Autodesk Fusion 360 part; units mm, degrees
(part 2 of 5)
  spline S37 degree 5 poles (9.6613, 25.5009) (9.6619, 25.504) (9.6641, 25.5157) (9.6678, 25.5361) (9.673, 25.5652) (9.6795, 25.6029) (9.6866, 25.6464) (9.6934, 25.69) (9.6999, 25.7337) (9.7061, 25.7775) (9.7119, 25.8213) (9.7174, 25.8653) (9.7226, 25.9094) (9.7275, 25.9535) (9.7322, 25.9977) (9.7365, 26.042) (9.7407, 26.0863) (9.7445, 26.1308) (9.7481, 26.1753) (9.7514, 26.2199) (9.7545, 26.2645) (9.7573, 26.3092) (9.7599, 26.354) (9.7623, 26.3988) (9.7644, 26.4437) (9.7663, 26.4886) (9.7679, 26.5336) (9.7694, 26.5787) (9.7706, 26.6238) (9.7715, 26.669) (9.7723, 26.7142) (9.7728, 26.7595) (9.7732, 26.8048) (9.7733, 26.8502) (9.7732, 26.8956) (9.7729, 26.9411) (9.7724, 26.9866) (9.7716, 27.0321) (9.7707, 27.0777) (9.7696, 27.1234) (9.7683, 27.169) (9.7667, 27.2148) (9.765, 27.2605) (9.7631, 27.3063) (9.761, 27.3522) (9.7587, 27.3981) (9.7562, 27.444) (9.7535, 27.4899) (9.7506, 27.5359) (9.7476, 27.582) (9.7443, 27.628) (9.7409, 27.6741) (9.7373, 27.7202) (9.7335, 27.7664) (9.7295, 27.8126) (9.7254, 27.8588) (9.721, 27.9051) (9.7165, 27.9514) (9.7118, 27.9977) (9.7069, 28.044) (9.7019, 28.0904) (9.6967, 28.1368) (9.6923, 28.1739) (9.689, 28.2018) (9.6868, 28.2203) (9.6856, 28.2296) knots 0.13777296 0.13777296 0.13777296 0.13777296 0.13777296 0.13777296 0.14285714 0.15714286 0.17142857 0.18571429 0.2 0.21428571 0.22857143 0.24285714 0.25714286 0.27142857 0.28571429 0.3 0.31428571 0.32857143 0.34285714 0.35714286 0.37142857 0.38571429 0.4 0.41428571 0.42857143 0.44285714 0.45714286 0.47142857 0.48571429 0.5 0.51428571 0.52857143 0.54285714 0.55714286 0.57142857 0.58571429 0.6 0.61428571 0.62857143 0.64285714 0.65714286 0.67142857 0.68571429 0.7 0.71428571 0.72857143 0.74285714 0.75714286 0.77142857 0.78571429 0.8 0.81428571 0.82857143 0.84285714 0.85714286 0.87142857 0.88571429 0.9 0.91428571 0.92857143 0.94285714 0.95714286 0.97142857 0.98571429 1 1 1 1 1 1
  arc A19 (9.6856, 28.2296) -> (8.7571, 28.5313) centre (0, 0) ccw
  spline S38 degree 5 poles (8.7571, 28.5313) (8.7507, 28.5245) (8.738, 28.5108) (8.7189, 28.4902) (8.6936, 28.4627) (8.6621, 28.4282) (8.6308, 28.3937) (8.5996, 28.359) (8.5686, 28.3243) (8.5377, 28.2895) (8.507, 28.2547) (8.4765, 28.2197) (8.4461, 28.1847) (8.4159, 28.1496) (8.3859, 28.1144) (8.356, 28.0791) (8.3263, 28.0438) (8.2968, 28.0083) (8.2674, 27.9728) (8.2382, 27.9372) (8.2092, 27.9015) (8.1804, 27.8658) (8.1517, 27.8299) (8.1233, 27.794) (8.095, 27.758) (8.0669, 27.7219) (8.0389, 27.6857) (8.0112, 27.6494) (7.9837, 27.6131) (7.9563, 27.5766) (7.9291, 27.5401) (7.9022, 27.5035) (7.8754, 27.4668) (7.8488, 27.4301) (7.8224, 27.3932) (7.7963, 27.3563) (7.7703, 27.3192) (7.7445, 27.2821) (7.719, 27.2449) (7.6937, 27.2076) (7.6685, 27.1702) (7.6436, 27.1328) (7.619, 27.0952) (7.5945, 27.0576) (7.5703, 27.0198) (7.5463, 26.982) (7.5226, 26.9441) (7.4991, 26.906) (7.4758, 26.8679) (7.4528, 26.8297) (7.4301, 26.7914) (7.4076, 26.753) (7.3854, 26.7145) (7.3634, 26.6759) (7.3417, 26.6372) (7.3203, 26.5984) (7.2992, 26.5595) (7.2785, 26.5205) (7.258, 26.4813) (7.2379, 26.4421) (7.2181, 26.4027) (7.2012, 26.3683) (7.1883, 26.3418) (7.1794, 26.3231) (7.1742, 26.3123) (7.1729, 26.3095) knots -1 -1 -1 -1 -1 -1 -0.98571429 -0.97142857 -0.95714286 -0.94285714 -0.92857143 -0.91428571 -0.9 -0.88571429 -0.87142857 -0.85714286 -0.84285714 -0.82857143 -0.81428571 -0.8 -0.78571429 -0.77142857 -0.75714286 -0.74285714 -0.72857143 -0.71428571 -0.7 -0.68571429 -0.67142857 -0.65714286 -0.64285714 -0.62857143 -0.61428571 -0.6 -0.58571429 -0.57142857 -0.55714286 -0.54285714 -0.52857143 -0.51428571 -0.5 -0.48571429 -0.47142857 -0.45714286 -0.44285714 -0.42857143 -0.41428571 -0.4 -0.38571429 -0.37142857 -0.35714286 -0.34285714 -0.32857143 -0.31428571 -0.3 -0.28571429 -0.27142857 -0.25714286 -0.24285714 -0.22857143 -0.21428571 -0.2 -0.18571429 -0.17142857 -0.15714286 -0.14285714 -0.13777296 -0.13777296 -0.13777296 -0.13777296 -0.13777296 -0.13777296
  spline S39 degree 3 poles (6.941, 26.2019) (6.9661, 26.1952) (6.9924, 26.1935) (7.044, 26.2003) (7.0689, 26.2087) (7.1092, 26.2317) (7.1252, 26.2444) (7.1527, 26.2742) (7.1642, 26.2911) (7.1729, 26.3095) knots 0 0 0 0 0.007813 0.007813 0.015626 0.015626 0.021719 0.021719 0.027811 0.027811 0.027811 0.027811
  arc A20 (6.941, 26.2019) -> (6.1725, 26.3935) centre (0, 0) ccw
  spline S40 degree 3 poles (6.0183, 26.5974) (6.0171, 26.5714) (6.021, 26.5454) (6.0385, 26.4963) (6.052, 26.4737) (6.083, 26.4393) (6.0988, 26.4264) (6.1338, 26.4057) (6.1527, 26.3981) (6.1725, 26.3935) knots 0 0 0 0 0.007813 0.007813 0.015626 0.015626 0.021719 0.021719 0.027811 0.027811 0.027811 0.027811
  spline S41 degree 5 poles (6.0183, 26.5974) (6.0184, 26.6005) (6.0189, 26.6124) (6.0198, 26.6331) (6.0209, 26.6626) (6.0221, 26.7009) (6.0231, 26.745) (6.0238, 26.7891) (6.0241, 26.8332) (6.0241, 26.8774) (6.0237, 26.9217) (6.0231, 26.966) (6.0221, 27.0103) (6.0208, 27.0547) (6.0193, 27.0991) (6.0174, 27.1436) (6.0153, 27.1881) (6.013, 27.2326) (6.0103, 27.2772) (6.0074, 27.3218) (6.0043, 27.3665) (6.0009, 27.4111) (5.9972, 27.4558) (5.9933, 27.5005) (5.9891, 27.5453) (5.9847, 27.5901) (5.9801, 27.6348) (5.9752, 27.6797) (5.9702, 27.7245) (5.9648, 27.7694) (5.9593, 27.8143) (5.9535, 27.8592) (5.9475, 27.9041) (5.9413, 27.949) (5.9349, 27.994) (5.9283, 28.039) (5.9214, 28.084) (5.9144, 28.129) (5.9071, 28.174) (5.8997, 28.2191) (5.892, 28.2641) (5.8841, 28.3092) (5.8761, 28.3543) (5.8678, 28.3994) (5.8593, 28.4445) (5.8506, 28.4896) (5.8418, 28.5347) (5.8327, 28.5798) (5.8235, 28.625) (5.8141, 28.6701) (5.8044, 28.7153) (5.7946, 28.7605) (5.7846, 28.8056) (5.7744, 28.8508) (5.7641, 28.896) (5.7535, 28.9412) (5.7428, 28.9864) (5.7319, 29.0316) (5.7208, 29.0768) (5.7095, 29.122) (5.698, 29.1672) (5.6864, 29.2124) (5.677, 29.2486) (5.6698, 29.2758) (5.665, 29.2938) (5.6626, 29.3029) knots 0.13777296 0.13777296 0.13777296 0.13777296 0.13777296 0.13777296 0.14285714 0.15714286 0.17142857 0.18571429 0.2 0.21428571 0.22857143 0.24285714 0.25714286 0.27142857 0.28571429 0.3 0.31428571 0.32857143 0.34285714 0.35714286 0.37142857 0.38571429 0.4 0.41428571 0.42857143 0.44285714 0.45714286 0.47142857 0.48571429 0.5 0.51428571 0.52857143 0.54285714 0.55714286 0.57142857 0.58571429 0.6 0.61428571 0.62857143 0.64285714 0.65714286 0.67142857 0.68571429 0.7 0.71428571 0.72857143 0.74285714 0.75714286 0.77142857 0.78571429 0.8 0.81428571 0.82857143 0.84285714 0.85714286 0.87142857 0.88571429 0.9 0.91428571 0.92857143 0.94285714 0.95714286 0.97142857 0.98571429 1 1 1 1 1 1
  arc A21 (5.6626, 29.3029) -> (4.7011, 29.4724) centre (0, 0) ccw
  spline S42 degree 5 poles (4.7011, 29.4724) (4.6957, 29.4647) (4.685, 29.4494) (4.669, 29.4264) (4.6478, 29.3956) (4.6214, 29.3571) (4.5951, 29.3185) (4.5691, 29.2799) (4.5432, 29.2412) (4.5175, 29.2025) (4.4919, 29.1637) (4.4666, 29.1248) (4.4414, 29.0859) (4.4163, 29.0469) (4.3915, 29.0079) (4.3668, 28.9688) (4.3423, 28.9296) (4.318, 28.8904) (4.2939, 28.8512) (4.27, 28.8119) (4.2462, 28.7725) (4.2226, 28.7331) (4.1992, 28.6936) (4.176, 28.654) (4.153, 28.6144) (4.1302, 28.5748) (4.1076, 28.5351) (4.0852, 28.4953) (4.063, 28.4555) (4.0409, 28.4156) (4.0191, 28.3756) (3.9975, 28.3356) (3.9761, 28.2956) (3.9549, 28.2555) (3.9339, 28.2153) (3.9131, 28.1751) (3.8926, 28.1348) (3.8722, 28.0944) (3.8521, 28.054) (3.8322, 28.0136) (3.8125, 27.9731) (3.7931, 27.9325) (3.7739, 27.8919) (3.7549, 27.8512) (3.7362, 27.8104) (3.7177, 27.7696) (3.6995, 27.7288) (3.6815, 27.6879) (3.6638, 27.6469) (3.6463, 27.6058) (3.6291, 27.5647) (3.6122, 27.5236) (3.5955, 27.4824) (3.5792, 27.4411) (3.5631, 27.3997) (3.5473, 27.3583) (3.5318, 27.3169) (3.5167, 27.2753) (3.5019, 27.2337) (3.4875, 27.1921) (3.4733, 27.1503) (3.4613, 27.1139) (3.4523, 27.0858) (3.446, 27.0661) (3.4425, 27.0547) (3.4415, 27.0517) knots -1 -1 -1 -1 -1 -1 -0.98571429 -0.97142857 -0.95714286 -0.94285714 -0.92857143 -0.91428571 -0.9 -0.88571429 -0.87142857 -0.85714286 -0.84285714 -0.82857143 -0.81428571 -0.8 -0.78571429 -0.77142857 -0.75714286 -0.74285714 -0.72857143 -0.71428571 -0.7 -0.68571429 -0.67142857 -0.65714286 -0.64285714 -0.62857143 -0.61428571 -0.6 -0.58571429 -0.57142857 -0.55714286 -0.54285714 -0.52857143 -0.51428571 -0.5 -0.48571429 -0.47142857 -0.45714286 -0.44285714 -0.42857143 -0.41428571 -0.4 -0.38571429 -0.37142857 -0.35714286 -0.34285714 -0.32857143 -0.31428571 -0.3 -0.28571429 -0.27142857 -0.25714286 -0.24285714 -0.22857143 -0.21428571 -0.2 -0.18571429 -0.17142857 -0.15714286 -0.14285714 -0.13777296 -0.13777296 -0.13777296 -0.13777296 -0.13777296 -0.13777296
  spline S43 degree 3 poles (3.2268, 26.9129) (3.2527, 26.9098) (3.2789, 26.9117) (3.3291, 26.9256) (3.3526, 26.9374) (3.3892, 26.9658) (3.4033, 26.9806) (3.4265, 27.014) (3.4355, 27.0323) (3.4415, 27.0517) knots 0 0 0 0 0.007813 0.007813 0.015626 0.015626 0.021719 0.021719 0.027811 0.027811 0.027811 0.027811
  arc A22 (3.2268, 26.9129) -> (2.4392, 26.9956) centre (0, 0) ccw
  spline S44 degree 3 poles (2.2581, 27.1761) (2.2605, 27.1502) (2.268, 27.125) (2.2922, 27.0788) (2.3087, 27.0584) (2.3442, 27.0286) (2.3616, 27.018) (2.3991, 27.0024) (2.419, 26.9975) (2.4392, 26.9956) knots 0 0 0 0 0.007813 0.007813 0.015626 0.015626 0.021719 0.021719 0.027811 0.027811 0.027811 0.027811
  spline S45 degree 5 poles (2.2581, 27.1761) (2.2578, 27.1792) (2.2566, 27.1911) (2.2546, 27.2117) (2.2516, 27.2411) (2.2474, 27.2792) (2.2423, 27.3229) (2.2368, 27.3667) (2.231, 27.4105) (2.2248, 27.4542) (2.2183, 27.498) (2.2115, 27.5418) (2.2044, 27.5856) (2.1969, 27.6294) (2.1892, 27.6731) (2.1812, 27.7169) (2.1729, 27.7607) (2.1644, 27.8045) (2.1556, 27.8482) (2.1465, 27.892) (2.1372, 27.9358) (2.1276, 27.9795) (2.1177, 28.0233) (2.1076, 28.067) (2.0973, 28.1107) (2.0867, 28.1545) (2.0759, 28.1982) (2.0648, 28.2419) (2.0536, 28.2856) (2.042, 28.3293) (2.0303, 28.373) (2.0183, 28.4166) (2.0062, 28.4603) (1.9938, 28.5039) (1.9812, 28.5476) (1.9683, 28.5912) (1.9553, 28.6348) (1.942, 28.6784) (1.9286, 28.7219) (1.9149, 28.7655) (1.9011, 28.8091) (1.887, 28.8526) (1.8727, 28.8961) (1.8583, 28.9396) (1.8436, 28.9831) (1.8287, 29.0266) (1.8137, 29.07) (1.7984, 29.1135) (1.783, 29.1569) (1.7674, 29.2003) (1.7515, 29.2437) (1.7355, 29.287) (1.7194, 29.3304) (1.703, 29.3737) (1.6864, 29.417) (1.6697, 29.4603) (1.6528, 29.5036) (1.6357, 29.5468) (1.6184, 29.59) (1.6009, 29.6332) (1.5833, 29.6764) (1.5655, 29.7196) (1.5511, 29.7541) (1.5402, 29.7799) (1.5329, 29.7972) (1.5293, 29.8058) knots 0.13777296 0.13777296 0.13777296 0.13777296 0.13777296 0.13777296 0.14285714 0.15714286 0.17142857 0.18571429 0.2 0.21428571 0.22857143 0.24285714 0.25714286 0.27142857 0.28571429 0.3 0.31428571 0.32857143 0.34285714 0.35714286 0.37142857 0.38571429 0.4 0.41428571 0.42857143 0.44285714 0.45714286 0.47142857 0.48571429 0.5 0.51428571 0.52857143 0.54285714 0.55714286 0.57142857 0.58571429 0.6 0.61428571 0.62857143 0.64285714 0.65714286 0.67142857 0.68571429 0.7 0.71428571 0.72857143 0.74285714 0.75714286 0.77142857 0.78571429 0.8 0.81428571 0.82857143 0.84285714 0.85714286 0.87142857 0.88571429 0.9 0.91428571 0.92857143 0.94285714 0.95714286 0.97142857 0.98571429 1 1 1 1 1 1
  arc A23 (1.5293, 29.8058) -> (0.5536, 29.8399) centre (0, 0) ccw
  spline S46 degree 5 poles (0.5536, 29.8399) (0.5493, 29.8315) (0.5409, 29.8148) (0.5282, 29.7898) (0.5115, 29.7564) (0.4907, 29.7145) (0.4701, 29.6727) (0.4497, 29.6308) (0.4294, 29.5889) (0.4093, 29.547) (0.3894, 29.505) (0.3697, 29.463) (0.3502, 29.4209) (0.3308, 29.3789) (0.3116, 29.3368) (0.2927, 29.2946) (0.2739, 29.2524) (0.2552, 29.2102) (0.2368, 29.168) (0.2186, 29.1257) (0.2005, 29.0834) (0.1827, 29.0411) (0.165, 28.9987) (0.1475, 28.9564) (0.1303, 28.9139) (0.1132, 28.8715) (0.0963, 28.829) (0.0797, 28.7865) (0.0632, 28.744) (0.0469, 28.7014) (0.0309, 28.6588) (0.015, 28.6162) (-0.0006, 28.5736) (-0.016, 28.5309) (-0.0312, 28.4882) (-0.0462, 28.4455) (-0.0609, 28.4027) (-0.0754, 28.3599) (-0.0897, 28.3171) (-0.1038, 28.2743) (-0.1177, 28.2314) (-0.1313, 28.1886) (-0.1446, 28.1457) (-0.1578, 28.1027) (-0.1706, 28.0598) (-0.1833, 28.0168) (-0.1956, 27.9738) (-0.2077, 27.9308) (-0.2196, 27.8877) (-0.2312, 27.8446) (-0.2425, 27.8016) (-0.2535, 27.7584) (-0.2643, 27.7153) (-0.2747, 27.6721) (-0.2849, 27.629) (-0.2948, 27.5858) (-0.3043, 27.5426) (-0.3135, 27.4993) (-0.3224, 27.4561) (-0.3309, 27.4128) (-0.3391, 27.3695) (-0.3459, 27.3318) (-0.3509, 27.3027) (-0.3544, 27.2823) (-0.3563, 27.2705) (-0.3568, 27.2674) knots -1 -1 -1 -1 -1 -1 -0.98571429 -0.97142857 -0.95714286 -0.94285714 -0.92857143 -0.91428571 -0.9 -0.88571429 -0.87142857 -0.85714286 -0.84285714 -0.82857143 -0.81428571 -0.8 -0.78571429 -0.77142857 -0.75714286 -0.74285714 -0.72857143 -0.71428571 -0.7 -0.68571429 -0.67142857 -0.65714286 -0.64285714 -0.62857143 -0.61428571 -0.6 -0.58571429 -0.57142857 -0.55714286 -0.54285714 -0.52857143 -0.51428571 -0.5 -0.48571429 -0.47142857 -0.45714286 -0.44285714 -0.42857143 -0.41428571 -0.4 -0.38571429 -0.37142857 -0.35714286 -0.34285714 -0.32857143 -0.31428571 -0.3 -0.28571429 -0.27142857 -0.25714286 -0.24285714 -0.22857143 -0.21428571 -0.2 -0.18571429 -0.17142857 -0.15714286 -0.14285714 -0.13777296 -0.13777296 -0.13777296 -0.13777296 -0.13777296 -0.13777296
  spline S47 degree 3 poles (-0.5501, 27.1) (-0.5241, 27.1006) (-0.4984, 27.1062) (-0.4506, 27.1269) (-0.429, 27.1419) (-0.3967, 27.1751) (-0.3848, 27.1917) (-0.3665, 27.228) (-0.3602, 27.2474) (-0.3568, 27.2674) knots 0 0 0 0 0.007813 0.007813 0.015626 0.015626 0.021719 0.021719 0.027811 0.027811 0.027811 0.027811
  arc A24 (-0.5501, 27.1) -> (-1.3416, 27.0724) centre (0, 0) ccw
  spline S48 degree 3 poles (-1.5461, 27.2259) (-1.5401, 27.2006) (-1.5292, 27.1766) (-1.4988, 27.1343) (-1.4796, 27.1163) (-1.4403, 27.0918) (-1.4215, 27.0837) (-1.3822, 27.0735) (-1.3619, 27.0714) (-1.3416, 27.0724) knots 0 0 0 0 0.007813 0.007813 0.015626 0.015626 0.021719 0.021719 0.027811 0.027811 0.027811 0.027811
  spline S49 degree 5 poles (-1.5461, 27.2259) (-1.5468, 27.2289) (-1.5496, 27.2405) (-1.5545, 27.2607) (-1.5615, 27.2893) (-1.571, 27.3265) (-1.5821, 27.3691) (-1.5937, 27.4117) (-1.6055, 27.4542) (-1.6177, 27.4967) (-1.6302, 27.5391) (-1.6431, 27.5815) (-1.6563, 27.6239) (-1.6697, 27.6662) (-1.6834, 27.7085) (-1.6975, 27.7507) (-1.7117, 27.7929) (-1.7263, 27.8351) (-1.7411, 27.8772) (-1.7562, 27.9193) (-1.7715, 27.9613) (-1.7871, 28.0033) (-1.803, 28.0453) (-1.8191, 28.0872) (-1.8354, 28.129) (-1.852, 28.1709) (-1.8687, 28.2127) (-1.8858, 28.2544) (-1.903, 28.2961) (-1.9205, 28.3378) (-1.9382, 28.3794) (-1.9561, 28.421) (-1.9743, 28.4625) (-1.9926, 28.504) (-2.0112, 28.5455) (-2.03, 28.5869) (-2.0489, 28.6282) (-2.0681, 28.6696) (-2.0875, 28.7108) (-2.1071, 28.7521) (-2.1269, 28.7933) (-2.1469, 28.8344) (-2.1671, 28.8755) (-2.1874, 28.9166) (-2.208, 28.9576) (-2.2288, 28.9986) (-2.2497, 29.0395) (-2.2709, 29.0804) (-2.2922, 29.1213) (-2.3137, 29.1621) (-2.3354, 29.2028) (-2.3573, 29.2436) (-2.3794, 29.2842) (-2.4016, 29.3248) (-2.424, 29.3654) (-2.4466, 29.406) (-2.4694, 29.4464) (-2.4924, 29.4869) (-2.5155, 29.5273) (-2.5388, 29.5676) (-2.5623, 29.6079) (-2.5859, 29.6482) (-2.605, 29.6804) (-2.6193, 29.7045) (-2.6289, 29.7205) (-2.6338, 29.7286) knots 0.13777296 0.13777296 0.13777296 0.13777296 0.13777296 0.13777296 0.14285714 0.15714286 0.17142857 0.18571429 0.2 0.21428571 0.22857143 0.24285714 0.25714286 0.27142857 0.28571429 0.3 0.31428571 0.32857143 0.34285714 0.35714286 0.37142857 0.38571429 0.4 0.41428571 0.42857143 0.44285714 0.45714286 0.47142857 0.48571429 0.5 0.51428571 0.52857143 0.54285714 0.55714286 0.57142857 0.58571429 0.6 0.61428571 0.62857143 0.64285714 0.65714286 0.67142857 0.68571429 0.7 0.71428571 0.72857143 0.74285714 0.75714286 0.77142857 0.78571429 0.8 0.81428571 0.82857143 0.84285714 0.85714286 0.87142857 0.88571429 0.9 0.91428571 0.92857143 0.94285714 0.95714286 0.97142857 0.98571429 1 1 1 1 1 1
  arc A25 (-2.6338, 29.7286) -> (-3.6047, 29.6265) centre (0, 0) ccw
  spline S50 degree 5 poles (-3.6047, 29.6265) (-3.6078, 29.6177) (-3.6138, 29.5999) (-3.6229, 29.5734) (-3.6348, 29.538) (-3.6496, 29.4937) (-3.6641, 29.4494) (-3.6785, 29.405) (-3.6928, 29.3607) (-3.7068, 29.3164) (-3.7207, 29.2721) (-3.7343, 29.2277) (-3.7478, 29.1834) (-3.7611, 29.139) (-3.7743, 29.0946) (-3.7872, 29.0502) (-3.8, 29.0059) (-3.8125, 28.9615) (-3.8249, 28.9171) (-3.8371, 28.8727) (-3.8491, 28.8283) (-3.8609, 28.7839) (-3.8725, 28.7395) (-3.8838, 28.6951) (-3.895, 28.6507) (-3.906, 28.6063) (-3.9168, 28.5619) (-3.9274, 28.5175) (-3.9378, 28.473) (-3.948, 28.4286) (-3.958, 28.3842) (-3.9677, 28.3398) (-3.9772, 28.2954) (-3.9866, 28.251) (-3.9957, 28.2066) (-4.0046, 28.1622) (-4.0132, 28.1178) (-4.0217, 28.0734) (-4.0299, 28.0291) (-4.0378, 27.9847) (-4.0456, 27.9403) (-4.0531, 27.896) (-4.0603, 27.8516) (-4.0674, 27.8073) (-4.0741, 27.7629) (-4.0807, 27.7186) (-4.0869, 27.6743) (-4.0929, 27.63) (-4.0987, 27.5858) (-4.1041, 27.5415) (-4.1093, 27.4972) (-4.1143, 27.453) (-4.1189, 27.4088) (-4.1233, 27.3646) (-4.1273, 27.3204) (-4.1311, 27.2763) (-4.1345, 27.2322) (-4.1376, 27.1881) (-4.1404, 27.144) (-4.1428, 27.1) (-4.1449, 27.0559) (-4.1464, 27.0176) (-4.1473, 26.9881) (-4.1479, 26.9674) (-4.1482, 26.9555) (-4.1483, 26.9524) knots -1 -1 -1 -1 -1 -1 -0.98571429 -0.97142857 -0.95714286 -0.94285714 -0.92857143 -0.91428571 -0.9 -0.88571429 -0.87142857 -0.85714286 -0.84285714 -0.82857143 -0.81428571 -0.8 -0.78571429 -0.77142857 -0.75714286 -0.74285714 -0.72857143 -0.71428571 -0.7 -0.68571429 -0.67142857 -0.65714286 -0.64285714 -0.62857143 -0.61428571 -0.6 -0.58571429 -0.57142857 -0.55714286 -0.54285714 -0.52857143 -0.51428571 -0.5 -0.48571429 -0.47142857 -0.45714286 -0.44285714 -0.42857143 -0.41428571 -0.4 -0.38571429 -0.37142857 -0.35714286 -0.34285714 -0.32857143 -0.31428571 -0.3 -0.28571429 -0.27142857 -0.25714286 -0.24285714 -0.22857143 -0.21428571 -0.2 -0.18571429 -0.17142857 -0.15714286 -0.14285714 -0.13777296 -0.13777296 -0.13777296 -0.13777296 -0.13777296 -0.13777296
  spline S51 degree 3 poles (-4.3164, 26.7597) (-4.2906, 26.7639) (-4.266, 26.773) (-4.2216, 26.8002) (-4.2022, 26.818) (-4.1748, 26.8554) (-4.1654, 26.8735) (-4.1523, 26.912) (-4.1487, 26.9321) (-4.1483, 26.9524) knots 0 0 0 0 0.007813 0.007813 0.015626 0.015626 0.021719 0.021719 0.027811 0.027811 0.027811 0.027811
  arc A26 (-4.3164, 26.7597) -> (-5.0963, 26.6222) centre (0, 0) ccw
  spline S52 degree 3 poles (-5.3202, 26.7458) (-5.3107, 26.7215) (-5.2965, 26.6993) (-5.2606, 26.6617) (-5.2391, 26.6465) (-5.1967, 26.6277) (-5.177, 26.6223) (-5.1367, 26.6176) (-5.1163, 26.6184) (-5.0963, 26.6222) knots 0 0 0 0 0.007813 0.007813 0.015626 0.015626 0.021719 0.021719 0.027811 0.027811 0.027811 0.027811
  spline S53 degree 5 poles (-5.3202, 26.7458) (-5.3213, 26.7487) (-5.3257, 26.7598) (-5.3333, 26.779) (-5.3443, 26.8064) (-5.3588, 26.8419) (-5.3758, 26.8825) (-5.3931, 26.9231) (-5.4108, 26.9636) (-5.4288, 27.004) (-5.4471, 27.0442) (-5.4657, 27.0844) (-5.4846, 27.1246) (-5.5039, 27.1646) (-5.5233, 27.2046) (-5.5431, 27.2444) (-5.5631, 27.2842) (-5.5834, 27.324) (-5.6039, 27.3636) (-5.6247, 27.4032) (-5.6458, 27.4427) (-5.667, 27.4821) (-5.6886, 27.5214) (-5.7103, 27.5607) (-5.7323, 27.5999) (-5.7546, 27.639) (-5.777, 27.678) (-5.7997, 27.717) (-5.8226, 27.7559) (-5.8457, 27.7947) (-5.869, 27.8335) (-5.8925, 27.8721) (-5.9163, 27.9107) (-5.9402, 27.9493) (-5.9644, 27.9877) (-5.9887, 28.0261) (-6.0133, 28.0645) (-6.038, 28.1027) (-6.063, 28.1409) (-6.0881, 28.179) (-6.1134, 28.2171) (-6.139, 28.255) (-6.1647, 28.2929) (-6.1906, 28.3308) (-6.2167, 28.3685) (-6.2429, 28.4062) (-6.2694, 28.4438) (-6.296, 28.4814) (-6.3228, 28.5189) (-6.3498, 28.5563) (-6.377, 28.5936) (-6.4043, 28.6309) (-6.4318, 28.6681) (-6.4595, 28.7052) (-6.4873, 28.7423) (-6.5154, 28.7793) (-6.5435, 28.8162) (-6.5719, 28.8531) (-6.6004, 28.8898) (-6.6291, 28.9266) (-6.658, 28.9632) (-6.687, 28.9998) (-6.7103, 29.029) (-6.7279, 29.0508) (-6.7397, 29.0654) (-6.7455, 29.0727) knots 0.13777296 0.13777296 0.13777296 0.13777296 0.13777296 0.13777296 0.14285714 0.15714286 0.17142857 0.18571429 0.2 0.21428571 0.22857143 0.24285714 0.25714286 0.27142857 0.28571429 0.3 0.31428571 0.32857143 0.34285714 0.35714286 0.37142857 0.38571429 0.4 0.41428571 0.42857143 0.44285714 0.45714286 0.47142857 0.48571429 0.5 0.51428571 0.52857143 0.54285714 0.55714286 0.57142857 0.58571429 0.6 0.61428571 0.62857143 0.64285714 0.65714286 0.67142857 0.68571429 0.7 0.71428571 0.72857143 0.74285714 0.75714286 0.77142857 0.78571429 0.8 0.81428571 0.82857143 0.84285714 0.85714286 0.87142857 0.88571429 0.9 0.91428571 0.92857143 0.94285714 0.95714286 0.97142857 0.98571429 1 1 1 1 1 1
  arc A27 (-6.7455, 29.0727) -> (-7.6928, 28.8365) centre (0, 0) ccw
  spline S54 degree 5 poles (-7.6928, 28.8365) (-7.6946, 28.8273) (-7.6982, 28.8089) (-7.7034, 28.7814) (-7.7103, 28.7446) (-7.7188, 28.6987) (-7.727, 28.6528) (-7.7351, 28.6069) (-7.743, 28.5611) (-7.7508, 28.5152) (-7.7583, 28.4694) (-7.7657, 28.4235) (-7.7729, 28.3777) (-7.7799, 28.332) (-7.7867, 28.2862) (-7.7934, 28.2405) (-7.7998, 28.1947) (-7.8061, 28.149) (-7.8122, 28.1034) (-7.818, 28.0577) (-7.8237, 28.0121) (-7.8292, 27.9665) (-7.8345, 27.9209) (-7.8396, 27.8753) (-7.8445, 27.8298) (-7.8493, 27.7843) (-7.8538, 27.7388) (-7.8581, 27.6933) (-7.8622, 27.6479) (-7.8661, 27.6025) (-7.8698, 27.5571) (-7.8732, 27.5118) (-7.8765, 27.4665) (-7.8796, 27.4212) (-7.8824, 27.376) (-7.885, 27.3308) (-7.8874, 27.2856) (-7.8896, 27.2405) (-7.8915, 27.1954) (-7.8933, 27.1504) (-7.8947, 27.1054) (-7.896, 27.0604) (-7.897, 27.0155) (-7.8978, 26.9706) (-7.8983, 26.9257) (-7.8986, 26.881) (-7.8987, 26.8362) (-7.8985, 26.7915) (-7.898, 26.7469) (-7.8972, 26.7023) (-7.8962, 26.6577) (-7.8949, 26.6132) (-7.8934, 26.5688) (-7.8916, 26.5245) (-7.8894, 26.4801) (-7.887, 26.4359) (-7.8843, 26.3917) (-7.8812, 26.3476) (-7.8778, 26.3036) (-7.874, 26.2597) (-7.87, 26.2158) (-7.8661, 26.1776) (-7.863, 26.1483) (-7.8607, 26.1277) (-7.8593, 26.1159) (-7.8589, 26.1128) knots -1 -1 -1 -1 -1 -1 -0.98571429 -0.97142857 -0.95714286 -0.94285714 -0.92857143 -0.91428571 -0.9 -0.88571429 -0.87142857 -0.85714286 -0.84285714 -0.82857143 -0.81428571 -0.8 -0.78571429 -0.77142857 -0.75714286 -0.74285714 -0.72857143 -0.71428571 -0.7 -0.68571429 -0.67142857 -0.65714286 -0.64285714 -0.62857143 -0.61428571 -0.6 -0.58571429 -0.57142857 -0.55714286 -0.54285714 -0.52857143 -0.51428571 -0.5 -0.48571429 -0.47142857 -0.45714286 -0.44285714 -0.42857143 -0.41428571 -0.4 -0.38571429 -0.37142857 -0.35714286 -0.34285714 -0.32857143 -0.31428571 -0.3 -0.28571429 -0.27142857 -0.25714286 -0.24285714 -0.22857143 -0.21428571 -0.2 -0.18571429 -0.17142857 -0.15714286 -0.14285714 -0.13777296 -0.13777296 -0.13777296 -0.13777296 -0.13777296 -0.13777296
  spline S55 degree 3 poles (-7.9986, 25.8986) (-7.9737, 25.9063) (-7.9506, 25.9187) (-7.9104, 25.9519) (-7.8937, 25.9722) (-7.8718, 26.013) (-7.8649, 26.0323) (-7.8573, 26.0722) (-7.8566, 26.0926) (-7.8589, 26.1128) knots 0 0 0 0 0.007813 0.007813 0.015626 0.015626 0.021719 0.021719 0.027811 0.027811 0.027811 0.027811
  arc A28 (-7.9986, 25.8986) -> (-8.7518, 25.6538) centre (0, 0) ccw
  spline S56 degree 3 poles (-8.9907, 25.745) (-8.9779, 25.7223) (-8.9608, 25.7024) (-8.92, 25.6701) (-8.8966, 25.6581) (-8.852, 25.6453) (-8.8318, 25.6427) (-8.7911, 25.6437) (-8.771, 25.6473) (-8.7518, 25.6538) knots 0 0 0 0 0.007813 0.007813 0.015626 0.015626 0.021719 0.021719 0.027811 0.027811 0.027811 0.027811
  spline S57 degree 5 poles (-8.9907, 25.745) (-8.9922, 25.7478) (-8.9981, 25.7581) (-9.0083, 25.7762) (-9.023, 25.8017) (-9.0423, 25.8349) (-9.0648, 25.8728) (-9.0876, 25.9105) (-9.1107, 25.9481) (-9.1342, 25.9856) (-9.1579, 26.023) (-9.1819, 26.0602) (-9.2063, 26.0973) (-9.2309, 26.1342) (-9.2557, 26.1711) (-9.2808, 26.2078) (-9.3062, 26.2445) (-9.3318, 26.281) (-9.3577, 26.3174) (-9.3838, 26.3537) (-9.4101, 26.3898) (-9.4367, 26.4259) (-9.4635, 26.4619) (-9.4905, 26.4977) (-9.5177, 26.5335) (-9.5452, 26.5691) (-9.5728, 26.6047) (-9.6007, 26.6401) (-9.6288, 26.6754) (-9.6571, 26.7107) (-9.6855, 26.7458) (-9.7142, 26.7808) (-9.7431, 26.8157) (-9.7722, 26.8506) (-9.8015, 26.8853) (-9.8309, 26.9199) (-9.8606, 26.9545) (-9.8904, 26.9889) (-9.9204, 27.0232) (-9.9506, 27.0575) (-9.981, 27.0916) (-10.0116, 27.1257) (-10.0423, 27.1596) (-10.0732, 27.1935) (-10.1043, 27.2272) (-10.1355, 27.2609) (-10.167, 27.2945) (-10.1986, 27.328) (-10.2303, 27.3613) (-10.2623, 27.3946) (-10.2944, 27.4278) (-10.3266, 27.4609) (-10.359, 27.494) (-10.3916, 27.5269) (-10.4243, 27.5597) (-10.4572, 27.5924) (-10.4903, 27.6251) (-10.5235, 27.6576) (-10.5569, 27.6901) (-10.5904, 27.7224) (-10.6241, 27.7547) (-10.6579, 27.7869) (-10.6851, 27.8126) (-10.7055, 27.8318) (-10.7192, 27.8446) (-10.726, 27.851) knots 0.13777296 0.13777296 0.13777296 0.13777296 0.13777296 0.13777296 0.14285714 0.15714286 0.17142857 0.18571429 0.2 0.21428571 0.22857143 0.24285714 0.25714286 0.27142857 0.28571429 0.3 0.31428571 0.32857143 0.34285714 0.35714286 0.37142857 0.38571429 0.4 0.41428571 0.42857143 0.44285714 0.45714286 0.47142857 0.48571429 0.5 0.51428571 0.52857143 0.54285714 0.55714286 0.57142857 0.58571429 0.6 0.61428571 0.62857143 0.64285714 0.65714286 0.67142857 0.68571429 0.7 0.71428571 0.72857143 0.74285714 0.75714286 0.77142857 0.78571429 0.8 0.81428571 0.82857143 0.84285714 0.85714286 0.87142857 0.88571429 0.9 0.91428571 0.92857143 0.94285714 0.95714286 0.97142857 0.98571429 1 1 1 1 1 1
  arc A29 (-10.726, 27.851) -> (-11.6312, 27.4852) centre (0, 0) ccw
  spline S58 degree 5 poles (-11.6312, 27.4852) (-11.6317, 27.4759) (-11.6327, 27.4572) (-11.634, 27.4292) (-11.6358, 27.3918) (-11.6377, 27.3452) (-11.6395, 27.2986) (-11.6412, 27.252) (-11.6426, 27.2055) (-11.6439, 27.159) (-11.645, 27.1125) (-11.6459, 27.0662) (-11.6467, 27.0198) (-11.6472, 26.9735) (-11.6476, 26.9272) (-11.6478, 26.881) (-11.6479, 26.8348) (-11.6477, 26.7887) (-11.6474, 26.7426) (-11.6468, 26.6966) (-11.6461, 26.6506) (-11.6452, 26.6047) (-11.6441, 26.5588) (-11.6428, 26.513) (-11.6414, 26.4672) (-11.6397, 26.4215) (-11.6378, 26.3758) (-11.6358, 26.3302) (-11.6335, 26.2846) (-11.631, 26.2391) (-11.6284, 26.1937) (-11.6255, 26.1483) (-11.6224, 26.103) (-11.6192, 26.0578) (-11.6157, 26.0126) (-11.612, 25.9674) (-11.6081, 25.9224) (-11.6039, 25.8774) (-11.5996, 25.8325) (-11.595, 25.7876) (-11.5902, 25.7428) (-11.5852, 25.6981) (-11.58, 25.6535) (-11.5745, 25.6089) (-11.5688, 25.5645) (-11.5629, 25.5201) (-11.5567, 25.4758) (-11.5502, 25.4315) (-11.5436, 25.3874) (-11.5366, 25.3433) (-11.5294, 25.2994) (-11.522, 25.2555) (-11.5142, 25.2117) (-11.5063, 25.168) (-11.498, 25.1244) (-11.4894, 25.081) (-11.4806, 25.0376) (-11.4714, 24.9944) (-11.4619, 24.9512) (-11.4521, 24.9082) (-11.4419, 24.8654) (-11.4328, 24.8281) (-11.4256, 24.7995) (-11.4204, 24.7794) (-11.4174, 24.7679) (-11.4167, 24.7649) knots -1 -1 -1 -1 -1 -1 -0.98571429 -0.97142857 -0.95714286 -0.94285714 -0.92857143 -0.91428571 -0.9 -0.88571429 -0.87142857 -0.85714286 -0.84285714 -0.82857143 -0.81428571 -0.8 -0.78571429 -0.77142857 -0.75714286 -0.74285714 -0.72857143 -0.71428571 -0.7 -0.68571429 -0.67142857 -0.65714286 -0.64285714 -0.62857143 -0.61428571 -0.6 -0.58571429 -0.57142857 -0.55714286 -0.54285714 -0.52857143 -0.51428571 -0.5 -0.48571429 -0.47142857 -0.45714286 -0.44285714 -0.42857143 -0.41428571 -0.4 -0.38571429 -0.37142857 -0.35714286 -0.34285714 -0.32857143 -0.31428571 -0.3 -0.28571429 -0.27142857 -0.25714286 -0.24285714 -0.22857143 -0.21428571 -0.2 -0.18571429 -0.17142857 -0.15714286 -0.14285714 -0.13777296 -0.13777296 -0.13777296 -0.13777296 -0.13777296 -0.13777296
  spline S59 degree 3 poles (-11.5251, 24.5334) (-11.5016, 24.5444) (-11.4804, 24.56) (-11.4452, 24.5984) (-11.4315, 24.6208) (-11.4155, 24.6643) (-11.4114, 24.6843) (-11.4094, 24.7249) (-11.4115, 24.7452) (-11.4167, 24.7649) knots 0 0 0 0 0.007813 0.007813 0.015626 0.015626 0.021719 0.021719 0.027811 0.027811 0.027811 0.027811
  arc A30 (-11.5251, 24.5334) -> (-12.237, 24.1862) centre (0, 0) ccw
  spline S60 degree 3 poles (-12.4862, 24.2432) (-12.4704, 24.2225) (-12.4507, 24.2051) (-12.4057, 24.1788) (-12.3809, 24.1702) (-12.335, 24.1637) (-12.3146, 24.164) (-12.2745, 24.1706) (-12.2551, 24.177) (-12.237, 24.1862) knots 0 0 0 0 0.007813 0.007813 0.015626 0.015626 0.021719 0.021719 0.027811 0.027811 0.027811 0.027811
  spline S61 degree 5 poles (-12.4862, 24.2432) (-12.4881, 24.2457) (-12.4953, 24.2552) (-12.508, 24.2716) (-12.5261, 24.2949) (-12.5498, 24.325) (-12.5774, 24.3594) (-12.6052, 24.3936) (-12.6333, 24.4276) (-12.6618, 24.4615) (-12.6905, 24.4952) (-12.7195, 24.5287) (-12.7487, 24.562) (-12.7782, 24.5952) (-12.808, 24.6283) (-12.8379, 24.6611) (-12.8682, 24.6939) (-12.8986, 24.7265) (-12.9293, 24.7589) (-12.9602, 24.7912) (-12.9913, 24.8234) (-13.0226, 24.8554) (-13.0541, 24.8873) (-13.0859, 24.919) (-13.1178, 24.9506) (-13.15, 24.9821) (-13.1823, 25.0135) (-13.2148, 25.0447) (-13.2476, 25.0758) (-13.2805, 25.1067) (-13.3136, 25.1375) (-13.3469, 25.1682) (-13.3803, 25.1988) (-13.414, 25.2292) (-13.4478, 25.2595) (-13.4818, 25.2897) (-13.5159, 25.3198) (-13.5503, 25.3498) (-13.5848, 25.3796) (-13.6195, 25.4093) (-13.6543, 25.4389) (-13.6893, 25.4683) (-13.7245, 25.4977) (-13.7598, 25.5269) (-13.7953, 25.556) (-13.8309, 25.585) (-13.8667, 25.6139) (-13.9026, 25.6426) (-13.9387, 25.6713) (-13.975, 25.6998) (-14.0114, 25.7282) (-14.0479, 25.7565) (-14.0846, 25.7847) (-14.1215, 25.8128) (-14.1585, 25.8407) (-14.1956, 25.8685) (-14.2329, 25.8963) (-14.2703, 25.9239) (-14.3079, 25.9514) (-14.3455, 25.9788) (-14.3834, 26.006) (-14.4214, 26.0332) (-14.4518, 26.0548) (-14.4748, 26.071) (-14.4901, 26.0818) (-14.4977, 26.0871) knots 0.13777296 0.13777296 0.13777296 0.13777296 0.13777296 0.13777296 0.14285714 0.15714286 0.17142857 0.18571429 0.2 0.21428571 0.22857143 0.24285714 0.25714286 0.27142857 0.28571429 0.3 0.31428571 0.32857143 0.34285714 0.35714286 0.37142857 0.38571429 0.4 0.41428571 0.42857143 0.44285714 0.45714286 0.47142857 0.48571429 0.5 0.51428571 0.52857143 0.54285714 0.55714286 0.57142857 0.58571429 0.6 0.61428571 0.62857143 0.64285714 0.65714286 0.67142857 0.68571429 0.7 0.71428571 0.72857143 0.74285714 0.75714286 0.77142857 0.78571429 0.8 0.81428571 0.82857143 0.84285714 0.85714286 0.87142857 0.88571429 0.9 0.91428571 0.92857143 0.94285714 0.95714286 0.97142857 0.98571429 1 1 1 1 1 1
  arc A31 (-14.4977, 26.0871) -> (-15.3433, 25.599) centre (0, 0) ccw
  spline S62 degree 5 poles (-15.3433, 25.599) (-15.3424, 25.5897) (-15.3408, 25.571) (-15.3382, 25.5431) (-15.3347, 25.5059) (-15.3302, 25.4594) (-15.3255, 25.413) (-15.3206, 25.3666) (-15.3156, 25.3204) (-15.3104, 25.2742) (-15.305, 25.228) (-15.2995, 25.1819) (-15.2938, 25.1359) (-15.2879, 25.09) (-15.2818, 25.0441) (-15.2756, 24.9983) (-15.2692, 24.9526) (-15.2626, 24.9069) (-15.2559, 24.8614) (-15.2489, 24.8158) (-15.2418, 24.7704) (-15.2345, 24.7251) (-15.2271, 24.6798) (-15.2194, 24.6346) (-15.2116, 24.5894) (-15.2036, 24.5444) (-15.1954, 24.4994) (-15.187, 24.4546) (-15.1784, 24.4098) (-15.1696, 24.3651) (-15.1607, 24.3204) (-15.1515, 24.2759) (-15.1422, 24.2314) (-15.1326, 24.1871) (-15.1229, 24.1428) (-15.1129, 24.0987) (-15.1028, 24.0546) (-15.0925, 24.0106) (-15.0819, 23.9667) (-15.0711, 23.9229) (-15.0602, 23.8793) (-15.049, 23.8357) (-15.0376, 23.7922) (-15.026, 23.7489) (-15.0141, 23.7056) (-15.0021, 23.6625) (-14.9898, 23.6194) (-14.9772, 23.5765) (-14.9645, 23.5338) (-14.9515, 23.4911) (-14.9382, 23.4486) (-14.9247, 23.4062) (-14.911, 23.3639) (-14.897, 23.3217) (-14.8827, 23.2797) (-14.8682, 23.2379) (-14.8534, 23.1962) (-14.8383, 23.1546) (-14.8229, 23.1132) (-14.8072, 23.072) (-14.7912, 23.031) (-14.7769, 22.9954) (-14.7658, 22.968) (-14.7579, 22.9489) (-14.7534, 22.9379) (-14.7522, 22.935) knots -1 -1 -1 -1 -1 -1 -0.98571429 -0.97142857 -0.95714286 -0.94285714 -0.92857143 -0.91428571 -0.9 -0.88571429 -0.87142857 -0.85714286 -0.84285714 -0.82857143 -0.81428571 -0.8 -0.78571429 -0.77142857 -0.75714286 -0.74285714 -0.72857143 -0.71428571 -0.7 -0.68571429 -0.67142857 -0.65714286 -0.64285714 -0.62857143 -0.61428571 -0.6 -0.58571429 -0.57142857 -0.55714286 -0.54285714 -0.52857143 -0.51428571 -0.5 -0.48571429 -0.47142857 -0.45714286 -0.44285714 -0.42857143 -0.41428571 -0.4 -0.38571429 -0.37142857 -0.35714286 -0.34285714 -0.32857143 -0.31428571 -0.3 -0.28571429 -0.27142857 -0.25714286 -0.24285714 -0.22857143 -0.21428571 -0.2 -0.18571429 -0.17142857 -0.15714286 -0.14285714 -0.13777296 -0.13777296 -0.13777296 -0.13777296 -0.13777296 -0.13777296
  spline S63 degree 3 poles (-14.8274, 22.6906) (-14.8056, 22.7049) (-14.7867, 22.7232) (-14.7572, 22.7661) (-14.7468, 22.7903) (-14.737, 22.8356) (-14.7357, 22.856) (-14.7394, 22.8964) (-14.7443, 22.9162) (-14.7522, 22.935) knots 0 0 0 0 0.007813 0.007813 0.015626 0.015626 0.021719 0.021719 0.027811 0.027811 0.027811 0.027811
  arc A32 (-14.8274, 22.6906) -> (-15.4839, 22.2477) centre (0, 0) ccw
  spline S64 degree 3 poles (-15.7387, 22.2696) (-15.7202, 22.2513) (-15.6982, 22.2368) (-15.65, 22.217) (-15.6243, 22.2119) (-15.5779, 22.2119) (-15.5577, 22.215) (-15.519, 22.2271) (-15.5006, 22.2361) (-15.4839, 22.2477) knots 0 0 0 0 0.007813 0.007813 0.015626 0.015626 0.021719 0.021719 0.027811 0.027811 0.027811 0.027811
  spline S65 degree 5 poles (-15.7387, 22.2696) (-15.7409, 22.2718) (-15.7494, 22.2801) (-15.7642, 22.2946) (-15.7854, 22.3152) (-15.8131, 22.3417) (-15.8451, 22.3719) (-15.8775, 22.4019) (-15.9101, 22.4317) (-15.9429, 22.4613) (-15.976, 22.4906) (-16.0094, 22.5198) (-16.043, 22.5487) (-16.0769, 22.5775) (-16.1109, 22.6061) (-16.1452, 22.6345) (-16.1797, 22.6627) (-16.2143, 22.6907) (-16.2492, 22.7186) (-16.2843, 22.7463) (-16.3196, 22.7738) (-16.3551, 22.8011) (-16.3907, 22.8283) (-16.4266, 22.8553) (-16.4626, 22.8822) (-16.4988, 22.9089) (-16.5352, 22.9354) (-16.5718, 22.9618) (-16.6085, 22.988) (-16.6454, 23.0141) (-16.6825, 23.04) (-16.7197, 23.0658) (-16.7571, 23.0914) (-16.7947, 23.1168) (-16.8324, 23.1422) (-16.8702, 23.1673) (-16.9082, 23.1923) (-16.9464, 23.2172) (-16.9847, 23.242) (-17.0232, 23.2665) (-17.0618, 23.291) (-17.1006, 23.3153) (-17.1395, 23.3395) (-17.1785, 23.3635) (-17.2177, 23.3874) (-17.257, 23.4111) (-17.2965, 23.4347) (-17.3361, 23.4582) (-17.3758, 23.4816) (-17.4157, 23.5048) (-17.4557, 23.5278) (-17.4958, 23.5508) (-17.5361, 23.5735) (-17.5765, 23.5962) (-17.617, 23.6187) (-17.6577, 23.6411) (-17.6984, 23.6634) (-17.7393, 23.6855) (-17.7803, 23.7075) (-17.8215, 23.7294) (-17.8627, 23.7512) (-17.9041, 23.7728) (-17.9373, 23.79) (-17.9623, 23.8028) (-17.9789, 23.8113) (-17.9873, 23.8156) knots 0.13777296 0.13777296 0.13777296 0.13777296 0.13777296 0.13777296 0.14285714 0.15714286 0.17142857 0.18571429 0.2 0.21428571 0.22857143 0.24285714 0.25714286 0.27142857 0.28571429 0.3 0.31428571 0.32857143 0.34285714 0.35714286 0.37142857 0.38571429 0.4 0.41428571 0.42857143 0.44285714 0.45714286 0.47142857 0.48571429 0.5 0.51428571 0.52857143 0.54285714 0.55714286 0.57142857 0.58571429 0.6 0.61428571 0.62857143 0.64285714 0.65714286 0.67142857 0.68571429 0.7 0.71428571 0.72857143 0.74285714 0.75714286 0.77142857 0.78571429 0.8 0.81428571 0.82857143 0.84285714 0.85714286 0.87142857 0.88571429 0.9 0.91428571 0.92857143 0.94285714 0.95714286 0.97142857 0.98571429 1 1 1 1 1 1
  arc A33 (-17.9873, 23.8156) -> (-18.7566, 23.2145) centre (0, 0) ccw
  spline S66 degree 5 poles (-18.7566, 23.2145) (-18.7545, 23.2054) (-18.7503, 23.1871) (-18.7439, 23.1598) (-18.7352, 23.1235) (-18.7243, 23.0781) (-18.7131, 23.0328) (-18.7019, 22.9876) (-18.6904, 22.9424) (-18.6789, 22.8974) (-18.6671, 22.8525) (-18.6552, 22.8076) (-18.6432, 22.7628) (-18.6309, 22.7182) (-18.6186, 22.6736) (-18.606, 22.6291) (-18.5933, 22.5847) (-18.5805, 22.5404) (-18.5674, 22.4962) (-18.5542, 22.4521) (-18.5409, 22.4081) (-18.5273, 22.3642) (-18.5136, 22.3204) (-18.4998, 22.2767) (-18.4857, 22.2331) (-18.4715, 22.1896) (-18.4571, 22.1462) (-18.4426, 22.103) (-18.4279, 22.0598) (-18.413, 22.0167) (-18.3979, 21.9738) (-18.3826, 21.931) (-18.3672, 21.8882) (-18.3516, 21.8457) (-18.3357, 21.8032) (-18.3198, 21.7608) (-18.3036, 21.7186) (-18.2872, 21.6765) (-18.2706, 21.6345) (-18.2539, 21.5926) (-18.237, 21.5509) (-18.2198, 21.5093) (-18.2025, 21.4679) (-18.1849, 21.4265) (-18.1672, 21.3853) (-18.1492, 21.3443) (-18.1311, 21.3034) (-18.1127, 21.2627) (-18.0941, 21.2221) (-18.0753, 21.1816) (-18.0562, 21.1414) (-18.037, 21.1012) (-18.0175, 21.0613) (-17.9978, 21.0215) (-17.9778, 20.9819) (-17.9576, 20.9425) (-17.9371, 20.9032) (-17.9164, 20.8642) (-17.8954, 20.8254) (-17.8741, 20.7867) (-17.8525, 20.7483) (-17.8335, 20.715) (-17.8187, 20.6895) (-17.8082, 20.6716) (-17.8021, 20.6614) (-17.8005, 20.6587) knots -1 -1 -1 -1 -1 -1 -0.98571429 -0.97142857 -0.95714286 -0.94285714 -0.92857143 -0.91428571 -0.9 -0.88571429 -0.87142857 -0.85714286 -0.84285714 -0.82857143 -0.81428571 -0.8 -0.78571429 -0.77142857 -0.75714286 -0.74285714 -0.72857143 -0.71428571 -0.7 -0.68571429 -0.67142857 -0.65714286 -0.64285714 -0.62857143 -0.61428571 -0.6 -0.58571429 -0.57142857 -0.55714286 -0.54285714 -0.52857143 -0.51428571 -0.5 -0.48571429 -0.47142857 -0.45714286 -0.44285714 -0.42857143 -0.41428571 -0.4 -0.38571429 -0.37142857 -0.35714286 -0.34285714 -0.32857143 -0.31428571 -0.3 -0.28571429 -0.27142857 -0.25714286 -0.24285714 -0.22857143 -0.21428571 -0.2 -0.18571429 -0.17142857 -0.15714286 -0.14285714 -0.13777296 -0.13777296 -0.13777296 -0.13777296 -0.13777296 -0.13777296
  spline S67 degree 3 poles (-17.841, 20.4062) (-17.8214, 20.4234) (-17.8053, 20.4442) (-17.782, 20.4908) (-17.7751, 20.5161) (-17.7717, 20.5623) (-17.7733, 20.5827) (-17.7825, 20.6223) (-17.7902, 20.6412) (-17.8005, 20.6587) knots 0 0 0 0 0.007813 0.007813 0.015626 0.015626 0.021719 0.021719 0.027811 0.027811 0.027811 0.027811
  arc A34 (-17.841, 20.4062) -> (-18.4295, 19.8763) centre (0, 0) ccw
  spline S68 degree 3 poles (-18.6848, 19.8624) (-18.6639, 19.8469) (-18.6402, 19.8356) (-18.5897, 19.8227) (-18.5635, 19.8213) (-18.5176, 19.8277) (-18.498, 19.8336) (-18.4613, 19.851) (-18.4444, 19.8625) (-18.4295, 19.8763) knots 0 0 0 0 0.007813 0.007813 0.015626 0.015626 0.021719 0.021719 0.027811 0.027811 0.027811 0.027811
  spline S69 degree 5 poles (-18.6848, 19.8624) (-18.6874, 19.8643) (-18.6969, 19.8714) (-18.7136, 19.8837) (-18.7374, 19.9011) (-18.7686, 19.9235) (-18.8045, 19.949) (-18.8407, 19.9742) (-18.8771, 19.9991) (-18.9138, 20.0238) (-18.9507, 20.0483) (-18.9878, 20.0725) (-19.0251, 20.0965) (-19.0626, 20.1203) (-19.1003, 20.1439) (-19.1382, 20.1672) (-19.1762, 20.1903) (-19.2145, 20.2133) (-19.2529, 20.236) (-19.2915, 20.2586) (-19.3303, 20.2809) (-19.3692, 20.303) (-19.4083, 20.325) (-19.4476, 20.3468) (-19.487, 20.3683) (-19.5266, 20.3897) (-19.5663, 20.4109) (-19.6062, 20.432) (-19.6462, 20.4528) (-19.6864, 20.4735) (-19.7267, 20.494) (-19.7671, 20.5144) (-19.8077, 20.5345) (-19.8484, 20.5545) (-19.8893, 20.5743) (-19.9303, 20.594) (-19.9714, 20.6135) (-20.0127, 20.6328) (-20.0541, 20.652) (-20.0956, 20.6709) (-20.1373, 20.6898) (-20.179, 20.7085) (-20.2209, 20.727) (-20.2629, 20.7453) (-20.305, 20.7635) (-20.3473, 20.7816) (-20.3897, 20.7995) (-20.4321, 20.8172) (-20.4747, 20.8348) (-20.5174, 20.8522) (-20.5603, 20.8695) (-20.6032, 20.8866) (-20.6462, 20.9036) (-20.6894, 20.9204) (-20.7327, 20.9371) (-20.776, 20.9536) (-20.8195, 20.97) (-20.8631, 20.9862) (-20.9068, 21.0023) (-20.9505, 21.0182) (-20.9944, 21.034) (-21.0384, 21.0496) (-21.0737, 21.062) (-21.1002, 21.0713) (-21.1179, 21.0774) (-21.1267, 21.0805) knots 0.13777296 0.13777296 0.13777296 0.13777296 0.13777296 0.13777296 0.14285714 0.15714286 0.17142857 0.18571429 0.2 0.21428571 0.22857143 0.24285714 0.25714286 0.27142857 0.28571429 0.3 0.31428571 0.32857143 0.34285714 0.35714286 0.37142857 0.38571429 0.4 0.41428571 0.42857143 0.44285714 0.45714286 0.47142857 0.48571429 0.5 0.51428571 0.52857143 0.54285714 0.55714286 0.57142857 0.58571429 0.6 0.61428571 0.62857143 0.64285714 0.65714286 0.67142857 0.68571429 0.7 0.71428571 0.72857143 0.74285714 0.75714286 0.77142857 0.78571429 0.8 0.81428571 0.82857143 0.84285714 0.85714286 0.87142857 0.88571429 0.9 0.91428571 0.92857143 0.94285714 0.95714286 0.97142857 0.98571429 1 1 1 1 1 1
  arc A35 (-21.1267, 21.0805) -> (-21.8049, 20.3782) centre (0, 0) ccw
  spline S70 degree 5 poles (-21.8049, 20.3782) (-21.8016, 20.3694) (-21.7948, 20.352) (-21.7847, 20.3258) (-21.7711, 20.291) (-21.7539, 20.2476) (-21.7366, 20.2043) (-21.7191, 20.1611) (-21.7015, 20.118) (-21.6838, 20.075) (-21.6659, 20.0321) (-21.6479, 19.9893) (-21.6297, 19.9467) (-21.6114, 19.9041) (-21.5929, 19.8617) (-21.5743, 19.8194) (-21.5556, 19.7772) (-21.5366, 19.7351) (-21.5176, 19.6932) (-21.4984, 19.6513) (-21.479, 19.6096) (-21.4595, 19.568) (-21.4399, 19.5266) (-21.4201, 19.4852) (-21.4001, 19.444) (-21.38, 19.4029) (-21.3597, 19.362) (-21.3392, 19.3211) (-21.3187, 19.2804) (-21.2979, 19.2399) (-21.277, 19.1995) (-21.2559, 19.1592) (-21.2347, 19.119) (-21.2133, 19.079) (-21.1917, 19.0391) (-21.17, 18.9994) (-21.1481, 18.9599) (-21.126, 18.9204) (-21.1038, 18.8812) (-21.0814, 18.842) (-21.0588, 18.8031) (-21.036, 18.7643) (-21.0131, 18.7256) (-20.99, 18.6872) (-20.9666, 18.6488) (-20.9432, 18.6107) (-20.9195, 18.5727) (-20.8956, 18.5349) (-20.8715, 18.4973) (-20.8473, 18.4599) (-20.8228, 18.4227) (-20.7982, 18.3856) (-20.7733, 18.3488) (-20.7482, 18.3121) (-20.723, 18.2757) (-20.6975, 18.2394) (-20.6717, 18.2034) (-20.6457, 18.1677) (-20.6195, 18.1321) (-20.5931, 18.0968) (-20.5664, 18.0618) (-20.5429, 18.0315) (-20.5247, 18.0083) (-20.5118, 17.992) (-20.5044, 17.9827) (-20.5024, 17.9803) knots -1 -1 -1 -1 -1 -1 -0.98571429 -0.97142857 -0.95714286 -0.94285714 -0.92857143 -0.91428571 -0.9 -0.88571429 -0.87142857 -0.85714286 -0.84285714 -0.82857143 -0.81428571 -0.8 -0.78571429 -0.77142857 -0.75714286 -0.74285714 -0.72857143 -0.71428571 -0.7 -0.68571429 -0.67142857 -0.65714286 -0.64285714 -0.62857143 -0.61428571 -0.6 -0.58571429 -0.57142857 -0.55714286 -0.54285714 -0.52857143 -0.51428571 -0.5 -0.48571429 -0.47142857 -0.45714286 -0.44285714 -0.42857143 -0.41428571 -0.4 -0.38571429 -0.37142857 -0.35714286 -0.34285714 -0.32857143 -0.31428571 -0.3 -0.28571429 -0.27142857 -0.25714286 -0.24285714 -0.22857143 -0.21428571 -0.2 -0.18571429 -0.17142857 -0.15714286 -0.14285714 -0.13777296 -0.13777296 -0.13777296 -0.13777296 -0.13777296 -0.13777296
  spline S71 degree 3 poles (-20.5073, 17.7246) (-20.4903, 17.7443) (-20.4773, 17.7672) (-20.4607, 17.8166) (-20.4574, 17.8426) (-20.4604, 17.8889) (-20.4649, 17.9088) (-20.4796, 17.9467) (-20.4897, 17.9644) (-20.5024, 17.9803) knots 0 0 0 0 0.007813 0.007813 0.015626 0.015626 0.021719 0.021719 0.027811 0.027811 0.027811 0.027811
  arc A36 (-20.5073, 17.7246) -> (-21.0164, 17.1179) centre (0, 0) ccw
  spline S72 degree 3 poles (-21.2673, 17.0687) (-21.2445, 17.0562) (-21.2194, 17.0483) (-21.1676, 17.0426) (-21.1414, 17.0448) (-21.0969, 17.0576) (-21.0783, 17.0661) (-21.0444, 17.0885) (-21.0293, 17.1022) (-21.0164, 17.1179) knots 0 0 0 0 0.007813 0.007813 0.015626 0.015626 0.021719 0.021719 0.027811 0.027811 0.027811 0.027811
  spline S73 degree 5 poles (-21.2673, 17.0687) (-21.2701, 17.0702) (-21.2805, 17.0759) (-21.2987, 17.0858) (-21.3248, 17.0997) (-21.3587, 17.1175) (-21.3979, 17.1377) (-21.4372, 17.1577) (-21.4767, 17.1773) (-21.5165, 17.1967) (-21.5564, 17.2158) (-21.5965, 17.2346) (-21.6368, 17.2532) (-21.6773, 17.2715) (-21.7179, 17.2896) (-21.7586, 17.3074) (-21.7996, 17.325) (-21.8406, 17.3424) (-21.8818, 17.3596) (-21.9232, 17.3765) (-21.9647, 17.3933) (-22.0063, 17.4098) (-22.0481, 17.4261) (-22.09, 17.4422) (-22.1321, 17.458) (-22.1742, 17.4737) (-22.2165, 17.4892) (-22.2589, 17.5045) (-22.3015, 17.5196) (-22.3441, 17.5345) (-22.3869, 17.5492) (-22.4298, 17.5637) (-22.4728, 17.578) (-22.5159, 17.5921) (-22.5591, 17.606) (-22.6025, 17.6198) (-22.6459, 17.6334) (-22.6895, 17.6468) (-22.7331, 17.66) (-22.7769, 17.673) (-22.8207, 17.6859) (-22.8647, 17.6986) (-22.9088, 17.7111) (-22.9529, 17.7234) (-22.9972, 17.7356) (-23.0415, 17.7475) (-23.086, 17.7594) (-23.1305, 17.771) (-23.1751, 17.7825) (-23.2198, 17.7938) (-23.2646, 17.8049) (-23.3095, 17.8159) (-23.3545, 17.8267) (-23.3996, 17.8374) (-23.4448, 17.8479) (-23.49, 17.8582) (-23.5353, 17.8684) (-23.5808, 17.8784) (-23.6262, 17.8882) (-23.6718, 17.8979) (-23.7175, 17.9074) (-23.7632, 17.9168) (-23.7999, 17.9242) (-23.8274, 17.9296) (-23.8458, 17.9332) (-23.855, 17.935) knots 0.13777296 0.13777296 0.13777296 0.13777296 0.13777296 0.13777296 0.14285714 0.15714286 0.17142857 0.18571429 0.2 0.21428571 0.22857143 0.24285714 0.25714286 0.27142857 0.28571429 0.3 0.31428571 0.32857143 0.34285714 0.35714286 0.37142857 0.38571429 0.4 0.41428571 0.42857143 0.44285714 0.45714286 0.47142857 0.48571429 0.5 0.51428571 0.52857143 0.54285714 0.55714286 0.57142857 0.58571429 0.6 0.61428571 0.62857143 0.64285714 0.65714286 0.67142857 0.68571429 0.7 0.71428571 0.72857143 0.74285714 0.75714286 0.77142857 0.78571429 0.8 0.81428571 0.82857143 0.84285714 0.85714286 0.87142857 0.88571429 0.9 0.91428571 0.92857143 0.94285714 0.95714286 0.97142857 0.98571429 1 1 1 1 1 1
  arc A37 (-23.855, 17.935) -> (-24.4288, 17.1452) centre (0, 0) ccw
  spline S74 degree 5 poles (-24.4288, 17.1452) (-24.4243, 17.137) (-24.4152, 17.1206) (-24.4015, 17.0961) (-24.3831, 17.0636) (-24.3601, 17.023) (-24.3369, 16.9825) (-24.3136, 16.9421) (-24.2902, 16.9019) (-24.2667, 16.8618) (-24.243, 16.8218) (-24.2192, 16.782) (-24.1952, 16.7423) (-24.1712, 16.7027) (-24.147, 16.6633) (-24.1227, 16.624) (-24.0982, 16.5848) (-24.0737, 16.5458) (-24.0489, 16.5069) (-24.0241, 16.4681) (-23.9991, 16.4295) (-23.974, 16.391) (-23.9488, 16.3527) (-23.9234, 16.3145) (-23.8979, 16.2765) (-23.8723, 16.2386) (-23.8465, 16.2008) (-23.8206, 16.1633) (-23.7945, 16.1258) (-23.7683, 16.0885) (-23.742, 16.0514) (-23.7155, 16.0145) (-23.6889, 15.9777) (-23.6621, 15.941) (-23.6352, 15.9045) (-23.6082, 15.8682) (-23.581, 15.8321) (-23.5536, 15.7961) (-23.5261, 15.7603) (-23.4985, 15.7247) (-23.4707, 15.6893) (-23.4428, 15.654) (-23.4147, 15.6189) (-23.3864, 15.5841) (-23.358, 15.5494) (-23.3294, 15.5149) (-23.3007, 15.4806) (-23.2718, 15.4465) (-23.2428, 15.4126) (-23.2135, 15.3789) (-23.1841, 15.3454) (-23.1545, 15.3122) (-23.1248, 15.2791) (-23.0949, 15.2463) (-23.0648, 15.2137) (-23.0345, 15.1814) (-23.004, 15.1493) (-22.9733, 15.1175) (-22.9424, 15.086) (-22.9113, 15.0547) (-22.8799, 15.0237) (-22.8525, 14.997) (-22.8312, 14.9765) (-22.8162, 14.9622) (-22.8075, 14.9541) (-22.8053, 14.9519) knots -1 -1 -1 -1 -1 -1 -0.98571429 -0.97142857 -0.95714286 -0.94285714 -0.92857143 -0.91428571 -0.9 -0.88571429 -0.87142857 -0.85714286 -0.84285714 -0.82857143 -0.81428571 -0.8 -0.78571429 -0.77142857 -0.75714286 -0.74285714 -0.72857143 -0.71428571 -0.7 -0.68571429 -0.67142857 -0.65714286 -0.64285714 -0.62857143 -0.61428571 -0.6 -0.58571429 -0.57142857 -0.55714286 -0.54285714 -0.52857143 -0.51428571 -0.5 -0.48571429 -0.47142857 -0.45714286 -0.44285714 -0.42857143 -0.41428571 -0.4 -0.38571429 -0.37142857 -0.35714286 -0.34285714 -0.32857143 -0.31428571 -0.3 -0.28571429 -0.27142857 -0.25714286 -0.24285714 -0.22857143 -0.21428571 -0.2 -0.18571429 -0.17142857 -0.15714286 -0.14285714 -0.13777296 -0.13777296 -0.13777296 -0.13777296 -0.13777296 -0.13777296
  spline S75 degree 3 poles (-22.7746, 14.6981) (-22.7604, 14.72) (-22.7507, 14.7444) (-22.7412, 14.7956) (-22.7415, 14.8219) (-22.751, 14.8673) (-22.7581, 14.8864) (-22.7779, 14.9218) (-22.7905, 14.938) (-22.8053, 14.9519) knots 0 0 0 0 0.007813 0.007813 0.015626 0.015626 0.021719 0.021719 0.027811 0.027811 0.027811 0.027811
  arc A38 (-22.7746, 14.6981) -> (-23.1943, 14.0264) centre (0, 0) ccw
  spline S76 degree 3 poles (-23.4359, 13.9427) (-23.4115, 13.9336) (-23.3856, 13.9292) (-23.3335, 13.9308) (-23.3079, 13.9366) (-23.2655, 13.9555) (-23.2483, 13.9665) (-23.2179, 13.9934) (-23.2048, 14.0091) (-23.1943, 14.0264) knots 0 0 0 0 0.007813 0.007813 0.015626 0.015626 0.021719 0.021719 0.027811 0.027811 0.027811 0.027811